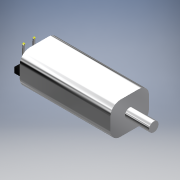
# Autodesk Inventor part: Motor
Saved by Autodesk Inventor 2018 (Build 220112000, 112)
## iProperties
Created: 2018-06-15
Part Number: Motor
Material: Aluminum 6061
Document SubType Name: Modeling
Designer: mmarkle
Density: 2.7 g/cm^3
Appearance: Aluminum - Flat
Author: mmarkle
Autodesk Inventor part; units mm, degrees
ref_plane "YZ Plane" through (0, 0, 0) normal (1, 0, 0) x (0, 1, 0)
ref_plane "XZ Plane" through (0, 0, 0) normal (0, 1, 0) x (-1, 0, 0)
sketch "Sketch1" plane through (0, 0, 0) normal (1, 0, 0) x (0, 1, 0)
  line L0 (-5.08, 6.096) -> (5.08, 6.096)
  line L1 (5.08, 6.096) -> (5.08, -6.096)
  line L2 (5.08, -6.096) -> (-5.08, -6.096)
  line L3 (-5.08, -6.096) -> (-5.08, 6.096)
  line L4 (-5.08, 6.096) -> (5.08, -6.096) construction
  line L5 (5.08, 6.096) -> (-5.08, -6.096) construction
  point P0 (0, 0)
  dimension "d0" = 10.16
  dimension "d1" = 12.192
  constraints: 12 end point, 2 midpoint, 2 parallel, 1 horizontal, 1 perpendicular
  measures "d0" distance of L1.end L2.end
  measures "d1" distance of L0.end L1.end
extrude "Extrusion1" add sketch "Sketch1" along normal blind 28.575
fillet "Fillet1" radius 3.175 4 edges at (14.2875, 5.08, 6.096) (14.2875, 5.08, -6.096) (14.2875, -5.08, -6.096) (14.2875, -5.08, 6.096)
sketch "Sketch2" plane through (28.575, 0, 0) normal (1, 0, 0) x (0, 0, -1)
  circle A0 centre (0, 0) radius 1.4986
  dimension "d5" = 2.9972
  constraints: 1 centre point, 1 coincident
  measures "d5" diameter of A0
extrude "Extrusion2" add sketch "Sketch2" along normal blind 7.62
sketch "Sketch3" plane through (0, 0, 0) normal (0, 0, 1) x (1, 0, 0)
  line L0 (0, -5.08) -> (0, -1.905) projected
  spline S0 degree 4 poles (0, -3.4925) (-0.3675, -3.5908) (-2.1702, -3.4732) (-3.8122, -3.0871) (-2.9446, -0.4736) (-3.4846, -0.0789) (-3.2353, 3.7565) knots 0 0 0 0 0 0.367245 0.503989 1 1 1 1 1
  point P0 (0, 0)
  point P1 (-1.2369, -3.4948)
  point P2 (-2.6438, -3.1804)
  point P3 (-3.1101, -2.7141)
  point P4 (-3.2352, -1.912)
  point P5 (-3.2353, -0.8631)
  constraints: 1 midpoint, 7 other
sketch "Sketch4" plane through (0, 0, 0) normal (-1, 0, 0) x (0, 0, 1)
  line L0 (-1.8758, -3.6581) -> (-1.3678, -3.6581)
  line L1 (-1.3678, -3.6581) -> (-1.3678, -3.2771)
  line L2 (-1.3678, -3.2771) -> (-1.8758, -3.2771)
  line L3 (-1.8758, -3.2771) -> (-1.8758, -3.6581)
  line L4 (-1.8758, -3.6581) -> (-1.3678, -3.2771) construction
  line L5 (-1.3678, -3.6581) -> (-1.8758, -3.2771) construction
  line L6 (2.921, -5.08) -> (-2.921, -5.08) projected
  line L7 (0, -5.08) -> (0, -4.0883)
  line L8 (1.8758, -3.6581) -> (1.3678, -3.6581)
  line L9 (1.3678, -3.6581) -> (1.3678, -3.2771)
  line L10 (1.3678, -3.2771) -> (1.8758, -3.2771)
  line L11 (1.8758, -3.2771) -> (1.8758, -3.6581)
  point P0 (0, 0)
  point P1 (-1.6218, -3.4676)
  dimension "d8" = 0.508
  dimension "d9" = 0.381
  constraints: 22 end point, 4 symmetric about line, 3 midpoint, 2 parallel, 1 horizontal, 1 perpendicular, 1 vertical
  measures "d8" distance of L2.end L1.end
  measures "d9" distance of L1.end L0.end
sweep "Sweep1" add profiles "Sketch4" path "Sketch3" path curves S0
ref_plane "Work Plane1" through (-3.175, 0, 0) normal (-1, 0, 0) x (0, 0, 1)
sketch "Sketch5" plane through (-3.175, 0, 0) normal (-1, 0, 0) x (0, 0, 1)
  line L0 (3.7701, -3.5576) -> (-3.7701, -3.5576)
  line L1 (-3.7701, -3.5576) -> (-3.7701, -1.8918)
  line L2 (-3.7701, -1.8918) -> (3.7701, -1.8918)
  line L3 (3.7701, -1.8918) -> (3.7701, -3.5576)
  line L4 (3.7701, -3.5576) -> (-3.7701, -1.8918) construction
  line L5 (-3.7701, -3.5576) -> (3.7701, -1.8918) construction
  point P0 (0, 0)
  point P1 (0, -2.7247)
  constraints: 12 end point, 2 midpoint, 2 parallel, 1 horizontal, 1 perpendicular
extrude "Extrusion3" add sketch "Sketch5" along normal mid plane 1.778
chamfer "Chamfer1" distance 0.1524 angle 45 8 edges at (-3.3921, 3.8095, 1.6218) (-3.2117, 3.7485, 1.8758) (-3.0312, 3.6874, 1.6218) (-3.2117, 3.7485, 1.3678) (-3.2117, 3.7485, -1.3678) (-3.0312, 3.6874, -1.6218) (-3.3921, 3.8095, -1.6218) (-3.2117, 3.7485, -1.8758)
body "Solid1"
